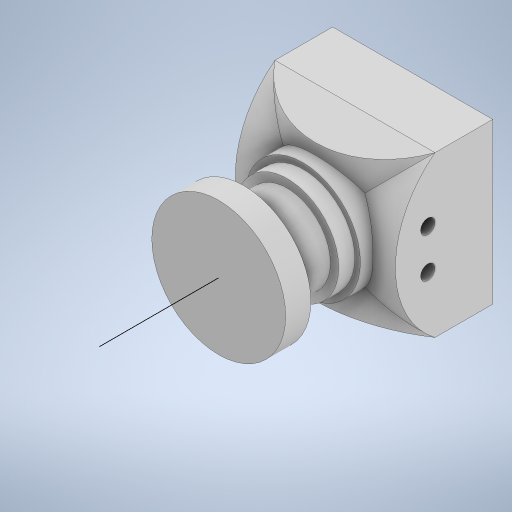
# Autodesk Inventor part: mini predator dummy camera
Saved by Autodesk Inventor 2023 (Build 270158000, 158)
## iProperties
Created: 2022-05-03
Part Number: mini predator dummy camera
Material: Generic
Document SubType Name: Modeling
Designer: Steven
Density: 1 g/cm^3
Appearance: Default
Author: Steven
Autodesk Inventor part; units mm, degrees
ref_plane "XZ Plane" through (0, 0, 0) normal (0, 1, 0) x (-1, 0, 0)
sketch "Sketch1" plane through (0, 0, 0) normal (0, 0, 1) x (1, 0, 0)
  line L0 (0, 0) -> (22.2, 0)
  line L1 (22.2, 0) -> (22.2, 22.2)
  line L2 (22.2, 22.2) -> (0, 22.2)
  line L3 (0, 22.2) -> (0, 0)
  dimension "d0" = 22.2
  dimension "d1" = 22.2
  constraints: 8 end point, 2 parallel, 1 horizontal, 1 perpendicular
  measures "d0" distance of L2.end L1.end
  measures "d1" distance of L1.end L0.end
extrude "Extrusion1" add sketch "Sketch1" along normal blind 8
sketch "Sketch2" plane through (0, 0, 8) normal (0, 0, 1) x (1, 0, 0)
  line L0 (0, 0) -> (22.2, 0) construction
  line L1 (22.2, 0) -> (22.2, 22.2) construction
  line L2 (22.2, 22.2) -> (0, 22.2) construction
  line L3 (0, 22.2) -> (0, 0) construction
  line L4 (22.2, 22.2) -> (0, 22.2) construction
  line L5 (11.1, 22.2) -> (11.1, 0) construction
  line L6 (0, 0) -> (22.2, 0) construction
  circle A0 centre (11.1, 11.1) radius 8
  dimension "d4" = 16
  constraints: 3 midpoint, 2 end point, 1 centre point
  measures "d4" diameter of A0
extrude "Extrusion2" add sketch "Sketch2" along normal blind 7.25
sketch "Sketch3" plane through (22.2, 0, 0) normal (1, 0, 0) x (0, 0, -1)
  line L0 (-15.25, 19.1) -> (-15.25, 3.1) construction
  line L1 (-15.25, 11.1) -> (0, 11.1) construction
  line L2 (0, 22.2) -> (0, 0) construction
  constraints: 2 end point, 2 midpoint
sketch "Sketch5" plane through (0, 0, 0) normal (0, -1, 0) x (1, 0, 0)
  line L0 (0, 0) -> (22.2, 0) construction
  line L1 (22.2, 0) -> (22.2, 8) construction
  line L2 (0, 8) -> (22.2, 8) construction
  line L3 (0, 0) -> (0, 8) construction
  line L4 (0, 8) -> (22.2, 8) construction
  line L5 (11.1, 8) -> (11.1, 13.5) construction
  arc A0 (22.2, 8) -> (0, 8) centre (11.1, -0.4509) ccw
  line L6 (0, 8) -> (22.2, 8)
  dimension "d9" = 5.5
  constraints: 4 end point, 3 point on circle, 1 centre point, 1 horizontal, 1 midpoint, 1 vertical
  measures "d9" distance of L5.start L5.end
extrude "Extrusion4" add sketch "Sketch5" against normal up to surface (22.2 mm away)
sketch "Sketch6" plane through (22.2, 0, 0) normal (1, 0, 0) x (0, 0, -1)
  line L0 (0, 0) -> (0, 22.2) construction
  line L1 (0, 22.2) -> (-8, 22.2) construction
  line L2 (-8, 0) -> (-8, 22.2) construction
  line L3 (0, 0) -> (-8, 0) construction
  line L4 (-8, 0) -> (-8, 22.2) construction
  line L5 (-8, 11.1) -> (-13.5, 11.1) construction
  line L6 (0, 22.2) -> (-8, 22.2) projected
  line L7 (0, 0) -> (-8, 0) projected
  arc A0 (-8, 22.2) -> (-8, 0) centre (0.4509, 11.1) ccw
  line L8 (-8, 22.2) -> (-8, 0)
  dimension "d12" = 5.5
  constraints: 4 end point, 3 point on circle, 1 centre point, 1 collinear, 1 horizontal, 1 midpoint
  measures "d12" distance of L5.start L5.end
extrude "Extrusion5" add sketch "Sketch6" against normal up to surface (22.2 mm away)
sketch "Sketch7" plane through (22.2, 0, 0) normal (1, 0, 0) x (0, 0, -1)
  line L0 (0, 0) -> (0, 22.2) construction
  line L1 (0, 22.2) -> (-8, 22.2) construction
  arc A0 (-8, 22.2) -> (-8, 0) centre (0.4509, 11.1) ccw construction
  line L2 (0, 0) -> (-8, 0) construction
  arc A1 (-8, 22.2) -> (-8, 0) centre (0.4509, 11.1) ccw construction
  line L3 (-13.5, 11.1) -> (0, 11.1) construction
  line L4 (0, 22.2) -> (0, 0) construction
  line L5 (-13.5, 11.1) -> (-13.5, 20.6) construction
  line L6 (-13.5, 11.1) -> (-13.5, 1.6) construction
  line L7 (0, 0) -> (-8, 0) projected
  line L8 (-13.5, 1.6) -> (-8, 0)
  line L9 (-8, 0) -> (-13.5, 0)
  line L10 (0, 0) -> (-8, 0) projected
  line L11 (-13.5, 0) -> (-13.5, 1.6)
  line L12 (0, 22.2) -> (-8, 22.2) projected
  line L13 (-13.5, 20.6) -> (-8, 22.2)
  line L14 (-8, 22.2) -> (-13.5, 22.2)
  line L15 (-13.5, 22.2) -> (-13.5, 20.6)
  dimension "d15" = 9.5
  constraints: 18 end point, 3 perpendicular, 2 collinear, 2 point on circle, 1 midpoint, 1 point on line, 1 symmetric about line, 1 tangent
  measures "d15" distance of L3.start L5.end
extrude "Extrusion6" cut sketch "Sketch7" against normal up to surface (22.2 mm away)
sketch "Sketch9" plane through (0, 0, 15.25) normal (0, 0, 1) x (1, 0, 0)
  arc A0 (17.7247, 6.5709) -> (17.7247, 15.8291) centre (11.2, 11.2) ccw projected
  arc A1 (17.7247, 15.8291) -> (16.9166, 16.7965) centre (11.2, 11.2) ccw projected
  arc A2 (16.9166, 16.7965) -> (16.7965, 16.9166) centre (11.2, 11.2) ccw projected
  arc A3 (16.7965, 16.9166) -> (15.8291, 17.7247) centre (11.2, 11.2) ccw projected
  arc A4 (15.8291, 17.7247) -> (6.5709, 17.7247) centre (11.2, 11.2) ccw projected
  arc A5 (6.5709, 17.7247) -> (5.6035, 16.9166) centre (11.2, 11.2) ccw projected
  arc A6 (5.6035, 16.9166) -> (5.4834, 16.7965) centre (11.2, 11.2) ccw projected
  arc A7 (5.4834, 16.7965) -> (4.6753, 15.8291) centre (11.2, 11.2) ccw projected
  arc A8 (4.6753, 15.8291) -> (4.6753, 6.5709) centre (11.2, 11.2) ccw projected
  arc A9 (4.6753, 6.5709) -> (5.4834, 5.6035) centre (11.2, 11.2) ccw projected
  arc A10 (5.4834, 5.6035) -> (5.6035, 5.4834) centre (11.2, 11.2) ccw projected
  arc A11 (5.6035, 5.4834) -> (6.5709, 4.6753) centre (11.2, 11.2) ccw projected
  arc A12 (6.5709, 4.6753) -> (15.8291, 4.6753) centre (11.2, 11.2) ccw projected
  arc A13 (15.8291, 4.6753) -> (16.7965, 5.4834) centre (11.2, 11.2) ccw projected
  arc A14 (16.7965, 5.4834) -> (16.9166, 5.6035) centre (11.2, 11.2) ccw projected
  arc A15 (16.9166, 5.6035) -> (17.7247, 6.5709) centre (11.2, 11.2) ccw projected
  circle A16 centre (11.2, 11.2) radius 7.1389
  point P0 (0, 0)
  constraints: 1 centre point, 1 coincident
extrude "Extrusion8" add sketch "Sketch9" along normal blind 2.25 contours A16
sketch "Sketch10" plane through (11.2, 11.2, 17.5) normal (0, 0, 1) x (1, 0, 0)
  circle A0 centre (0, 0) radius 8 projected
  circle A1 centre (0, 0) radius 6
  circle A2 centre (0, 0) radius 7
  point P0 (-11.2, -11.2)
  dimension "d25" = 2
  dimension "d36" = 1
  constraints: 2 centre point
  measures "d25" radial gap between concentric circles of A0 A1
  measures "d36" radial gap between concentric circles of A0 A2
extrude "Extrusion9" add sketch "Sketch10" along normal blind 6 contours A1
sketch "Sketch11" plane through (11.2, 11.2, 23.5) normal (0, 0, 1) x (1, 0, 0)
  circle A0 centre (0, 0) radius 6 projected
  circle A1 centre (0, 0) radius 9.28
  point P0 (-11.2, -11.2)
  dimension "d28" = 18.56
  constraints: 1 centre point, 1 coincident
  measures "d28" diameter of A1
extrude "Extrusion10" add sketch "Sketch11" along normal blind 3.5 contours A0 | A1
sketch "Sketch12" plane through (22.2, 0, 0) normal (1, 0, 0) x (0, 0, -1)
  line L0 (-27, 20.48) -> (-27, 1.92) construction
  line L1 (-27, 11.2) -> (0, 11.1) construction
  line L2 (0, 0) -> (0, 22.2) construction
  dimension "d31" = 27.0002
  constraints: 2 end point, 2 midpoint
  measures "d31" distance of L1.start L1.end
ref_plane "Work Plane2" through (11.2, 0, 0) normal (1, 0, 0) x (0, 1, 0)
sketch "Sketch17" plane through (0, 0, 0) normal (-1, 0, 0) x (0, 0, 1)
  line L0 (0, 22.2) -> (0, 0) construction
  line L1 (0, 0) -> (8, 0) construction
  arc A0 (8, 0) -> (8, 22.2) centre (-0.4509, 11.1) ccw construction
  line L2 (0, 22.2) -> (8, 22.2) construction
  line L3 (0, 22.2) -> (0, 0) construction
  line L4 (0, 11.1) -> (9, 11.1) construction
  line L5 (9, 11.1) -> (9, 8.35) construction
  line L6 (17.5, 17.2) -> (23.5, 17.2) construction
  line L7 (9, 11.1) -> (9, 13.85) construction
  circle A1 centre (9, 8.35) radius 1
  circle A2 centre (9, 13.85) radius 1
  dimension "d48" = 9
  dimension "d49" = 2.75
  dimension "d50" = 2
  dimension "d52" = 2.75
  dimension "d53" = 2
  constraints: 6 end point, 2 centre point, 2 coincident, 1 horizontal, 1 midpoint, 1 perpendicular, 1 symmetric about line
  measures "d48" distance of L4.start L4.end
  measures "d49" distance of L4.end L5.end
  measures "d50" diameter of A1
  measures "d52" distance of L4.end L7.end
  measures "d53" diameter of A2
extrude "Extrusion12" cut sketch "Sketch17" against normal through all
ref_plane "Work Plane4" through (11.1, 0, 0) normal (1, 0, 0) x (0, 0, -1)
sketch "Sketch18" plane through (11.1, 0, 0) normal (1, 0, 0) x (0, 0, -1)
  line L0 (0, 0) -> (0, 22.2) projected
  line L1 (0, 11.1) -> (-43.4569, 11.1)
  constraints: 2 end point, 1 horizontal, 1 midpoint
body "Solid1"
